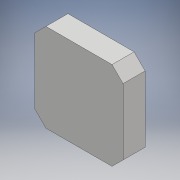
# Autodesk Inventor part: Plateau
Saved by Autodesk Inventor 2018 (Build 220112000, 112)
## iProperties
Created: 2018-03-19
Part Number: Plateau
Material: Générique
Document SubType Name: Modeling
Designer: Youri
Density: 1 g/cm^3
Appearance: Par défaut
Author: Youri
Autodesk Inventor part; units mm, degrees
ref_plane "YZ Plane" through (0, 0, 0) normal (1, 0, 0) x (0, 1, 0)
ref_plane "XZ Plane" through (0, 0, 0) normal (0, 1, 0) x (-1, 0, 0)
ref_plane "XY Plane" through (0, 0, 0) normal (0, 0, 1) x (1, 0, 0)
sketch "Esquisse1" plane through (0, 0, 0) normal (0, 1, 0) x (-1, 0, 0)
  line L0 (0, 0) -> (32, 0)
  line L1 (32, 0) -> (32, 32)
  line L2 (32, 32) -> (0, 32)
  line L3 (0, 32) -> (0, 0)
  dimension "d0" = 32
  dimension "d1" = 32
  constraints: 8 end point, 2 parallel, 1 horizontal, 1 perpendicular
  measures "d0" distance of L2.end L0.start
  measures "d1" distance of L1.end L2.end
extrude "Extrusion1" add sketch "Esquisse1" along normal blind 8
sketch "Esquisse2" plane through (0, 8, 0) normal (0, 1, 0) x (1, 0, 0)
  line L0 (-32, 0) -> (-32, -32) projected
  line L1 (-32, -30) -> (12, -30)
  line L2 (-32, -2) -> (0.5255, -2)
  line L3 (-30, -30) -> (-30, -2)
  line L4 (-2, -30) -> (-2, -2)
  line L5 (0, -32) -> (0, 0) projected
  line L6 (-32, -32) -> (0, -32) projected
  line L7 (0, 0) -> (-32, 0) projected
  circle A0 centre (-26, -26) radius 4
  circle A1 centre (-26, -16) radius 4
  circle A2 centre (-26, -6) radius 4
  circle A3 centre (-16, -26) radius 4
  circle A4 centre (-16, -16) radius 4
  circle A5 centre (-16, -6) radius 4
  circle A6 centre (-6, -26) radius 4
  circle A7 centre (-6, -16) radius 4
  circle A8 centre (-6, -6) radius 4
  dimension "d4" = 2
  dimension "d5" = 2
  dimension "d6" = 2
  dimension "d7" = 2
  dimension "d18" = 8
  dimension "d19" = 8
  dimension "d20" = 8
  dimension "d21" = 8
  dimension "d22" = 8
  dimension "d23" = 8
  dimension "d24" = 8
  dimension "d25" = 8
  dimension "d26" = 8
  dimension "d27" = 4
  dimension "d28" = 4
  dimension "d29" = 4
  dimension "d30" = 4
  dimension "d31" = 4
  dimension "d32" = 4
  dimension "d33" = 4
  dimension "d34" = 4
  dimension "d35" = 10
  dimension "d36" = 4
  dimension "d37" = 4
  dimension "d38" = 4
  dimension "d39" = 10
  dimension "d40" = 10
  dimension "d41" = 10
  dimension "d42" = 10
  dimension "d43" = 10
  dimension "d44" = 10
  dimension "d45" = 10
  constraints: 9 centre point, 8 end point, 6 point on line, 2 horizontal, 2 perpendicular, 1 other
  measures "d4" distance between parallel lines of L3 L0
  measures "d5" distance of the line from the sketch origin of L4
  measures "d6" distance between parallel lines of L6 L1
  measures "d7" distance between parallel lines of L7 L2
  measures "d18" diameter of A0
  measures "d19" diameter of A1
  measures "d20" diameter of A2
  measures "d21" diameter of A5
  measures "d22" diameter of A4
  measures "d23" diameter of A3
  measures "d24" diameter of A6
  measures "d25" diameter of A7
  measures "d26" diameter of A8
  measures "d27" distance from line of L1 A0.centre
  measures "d28" distance from line of L3 A0.centre
  measures "d29" distance from line of L2 A2.centre
  measures "d30" distance from line of L3 A2.centre
  measures "d31" distance from line of L1 A3.centre
  measures "d32" distance from line of L2 A5.centre
  measures "d33" distance from line of L2 A8.centre
  measures "d34" distance from line of L1 A6.centre
  measures "d35" distance of A7.centre A6.centre
  measures "d36" distance from line of L4 A7.centre
  measures "d37" distance from line of L4 A8.centre
  measures "d38" distance from line of L4 A6.centre
  measures "d39" distance of A4.centre A3.centre
  measures "d40" distance of A7.centre A4.centre
  measures "d41" distance of A6.centre A3.centre
  measures "d42" distance of A5.centre A4.centre
  measures "d43" distance of A8.centre A5.centre
  measures "d44" distance of A1.centre A0.centre
  measures "d45" distance of A4.centre A1.centre
extrude "Extrusion2" cut sketch "Esquisse2" against normal blind 6 contours A1 | A3 | A7 | A5 | A2 | A0 | A8 | A6 | A4
chamfer "Chanfrein1" distance 4 angle 45 4 edges at (0, 4, 32) (0, 4, 0) (-32, 4, 0) (-32, 4, 32)
chamfer "Chanfrein2" distance 1 angle 45 9 edges at (-30, 8, 26) (-30, 8, 16) (-30, 8, 6) (-20, 8, 6) (-20, 8, 16) (-20, 8, 26) (-10, 8, 16) (-10, 8, 26) (-10, 8, 6)
